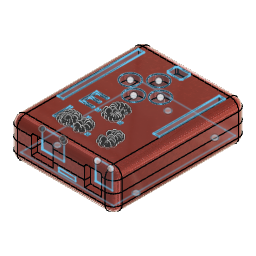
EdwinSolano_lab3_caja (Autodesk Fusion 360 design; units mm, degrees)
Autodesk Fusion 360 part; units mm, degrees
note: some values were not read from the file. Set by a fixed rule: which face or edge a step refers to.
sketch "sketch 1624" plane through (0, 0, 0) normal (0, 0, 1) x (1, 0, 0)
  line L0 (-54.34, 66.04) -> (-54.34, 0)
  line L1 (-54.34, 0) -> (-54.34, -3)
  line L2 (-54.34, -3) -> (-53.34, -3)
  line L3 (-53.34, -3) -> (0, -3)
  line L4 (0, -3) -> (1, -3)
  line L5 (1, -3) -> (1, 0)
  line L6 (1, 0) -> (1, 66.04)
  line L7 (1, 69.58) -> (1, 66.04)
  line L8 (-5.08, 69.58) -> (1, 69.58)
  line L9 (-5.08, 69.58) -> (-37.846, 69.58)
  line L10 (-54.34, 69.58) -> (-37.846, 69.58)
  line L11 (-54.34, 66.04) -> (-54.34, 69.58)
extrude "Extrude1" add sketch "sketch 1624" along normal blind 16.5 makes body 1
fillet "Fillet1" radius 1.5 11 edges at (-54.34, 33.29, 16.5) (-53.84, -3, 16.5) (-26.17, -3, 16.5) (1, 33.29, 16.5) (-26.67, 69.58, 16.5) (-54.34, 69.58, 8.25) (-54.34, -3, 8.25) (1, -3, 8.25) (-53.84, -3, 0) (-26.17, -3, 0) (-54.34, 33.29, 0) on bodies 1
fillet "Fillet2" radius 1.5 6 edges at (0.5607, -2.5607, 0.4393) (1, 34.04, 0) (1, 69.58, 7.5) (0.5607, 69.1407, 16.0607) (-53.9007, 69.1407, 0.4393) (-25.92, 69.58, 0) on bodies 1
shell "Shell1" thickness 3.6 outward yes removed faces 0 bodies 1
ref_plane "WorkPlane1" through (-26.67, 33.29, 8.25) normal (0, 0, 1) x (1, 0, 0)
split "Split1" by plane through (-26.67, 33.29, 8.25) normal (0, 0, 1) bodies 1 makes body 2 at (-35.3933, 21.6933, 20.1)
copy_body "Body->Comp1" bodies 2 removing the originals makes body 3 in component "parteArriba"
copy_body "Body->Comp2" bodies 1 removing the originals makes body 4 in component "parteAbajo"
sketch "sketch 1670" plane through (0, 0, 0) normal (0, -1, 0) x (1, 0, 0)
  spline S0 degree 3 poles (-31.5, 15.59) (-31.5, 15.7159) (-31.5248, 15.8406) (-31.5729, 15.9569) (-31.6211, 16.0735) (-31.6918, 16.1794) (-31.7809, 16.2686) (-31.8701, 16.3578) (-31.9759, 16.4286) (-32.0924, 16.4768) (-32.209, 16.5251) (-32.3339, 16.55) (-32.46, 16.55) knots -0.073178 -0.073178 -0.073178 -0.073178 -0.054906 -0.054906 -0.054906 -0.036606 -0.036606 -0.036606 -0.018305 -0.018305 -0.018305 0 0 0 0
  line L0 (-32.46, 16.55) -> (-43.58, 16.55)
  spline S1 degree 3 poles (-43.58, 16.55) (-43.7059, 16.55) (-43.8306, 16.5252) (-43.9469, 16.4771) (-44.0635, 16.4289) (-44.1694, 16.3582) (-44.2586, 16.2691) (-44.3478, 16.1799) (-44.4186, 16.0741) (-44.4668, 15.9576) (-44.5151, 15.841) (-44.54, 15.7161) (-44.54, 15.59) knots -0.073178 -0.073178 -0.073178 -0.073178 -0.054906 -0.054906 -0.054906 -0.036606 -0.036606 -0.036606 -0.018305 -0.018305 -0.018305 0 0 0 0
  line L1 (-44.54, 15.59) -> (-44.54, 15.49)
  line L2 (-44.54, 15.49) -> (-44.54, 5.84)
  line L3 (-44.54, 5.84) -> (-44.54, 5)
  line L4 (-31.5, 5) -> (-44.54, 5)
  line L5 (-31.5, 5) -> (-31.5, 5.84)
  line L6 (-31.5, 5.84) -> (-31.5, 15.49)
  line L7 (-31.5, 15.59) -> (-31.5, 15.49)
  arc A0 (-11.675, 16.5) -> (-12.675, 15.5) centre (-11.675, 15.5) ccw
  line L8 (-12.675, 15.5) -> (-12.675, 4.5)
  line L9 (-12.675, 4.5) -> (-2.675, 4.5)
  line L10 (-2.675, 4.5) -> (-2.675, 15.5)
  arc A1 (-2.675, 15.5) -> (-3.675, 16.5) centre (-3.675, 15.5) ccw
  line L11 (-3.675, 16.5) -> (-11.675, 16.5)
extrude "Extrude1'" cut sketch "sketch 1670" along normal up to surface (6.6 mm away) bodies 3 in component "parteArriba"
sketch "sketch 1744" plane through (0, 0, 0) normal (0, -1, 0) x (1, 0, 0)
  spline S0 degree 3 poles (-31.5, 15.59) (-31.5, 15.7159) (-31.5248, 15.8406) (-31.5729, 15.9569) (-31.6211, 16.0735) (-31.6918, 16.1794) (-31.7809, 16.2686) (-31.8701, 16.3578) (-31.9759, 16.4286) (-32.0924, 16.4768) (-32.209, 16.5251) (-32.3339, 16.55) (-32.46, 16.55) knots -0.073178 -0.073178 -0.073178 -0.073178 -0.054906 -0.054906 -0.054906 -0.036606 -0.036606 -0.036606 -0.018305 -0.018305 -0.018305 0 0 0 0
  line L0 (-32.46, 16.55) -> (-43.58, 16.55)
  spline S1 degree 3 poles (-43.58, 16.55) (-43.7059, 16.55) (-43.8306, 16.5252) (-43.9469, 16.4771) (-44.0635, 16.4289) (-44.1694, 16.3582) (-44.2586, 16.2691) (-44.3478, 16.1799) (-44.4186, 16.0741) (-44.4668, 15.9576) (-44.5151, 15.841) (-44.54, 15.7161) (-44.54, 15.59) knots -0.073178 -0.073178 -0.073178 -0.073178 -0.054906 -0.054906 -0.054906 -0.036606 -0.036606 -0.036606 -0.018305 -0.018305 -0.018305 0 0 0 0
  line L1 (-44.54, 15.59) -> (-44.54, 15.49)
  line L2 (-44.54, 15.49) -> (-44.54, 5.84)
  line L3 (-44.54, 5.84) -> (-44.54, 5)
  line L4 (-31.5, 5) -> (-44.54, 5)
  line L5 (-31.5, 5) -> (-31.5, 5.84)
  line L6 (-31.5, 5.84) -> (-31.5, 15.49)
  line L7 (-31.5, 15.59) -> (-31.5, 15.49)
  arc A0 (-11.675, 16.5) -> (-12.675, 15.5) centre (-11.675, 15.5) ccw
  line L8 (-12.675, 15.5) -> (-12.675, 4.5)
  line L9 (-12.675, 4.5) -> (-2.675, 4.5)
  line L10 (-2.675, 4.5) -> (-2.675, 15.5)
  arc A1 (-2.675, 15.5) -> (-3.675, 16.5) centre (-3.675, 15.5) ccw
  line L11 (-3.675, 16.5) -> (-11.675, 16.5)
extrude "Extrude1''" cut sketch "sketch 1744" along normal up to surface (6.6 mm away) bodies 4 in component "parteAbajo"
sketch "sketch 1818" plane through (0, 0, 20.1) normal (0, 0, 1) x (-1, 0, 0)
  line L0 (32.2, -62.7029) -> (32.2, -67.1171)
  line L1 (31.4071, -61.91) -> (32.2, -62.7029)
  line L2 (24.3729, -61.91) -> (31.4071, -61.91)
  line L3 (23.58, -62.7029) -> (24.3729, -61.91)
  line L4 (23.58, -67.1171) -> (23.58, -62.7029)
  line L5 (24.3729, -67.91) -> (23.58, -67.1171)
  line L6 (31.4071, -67.91) -> (24.3729, -67.91)
  line L7 (32.2, -67.1171) -> (31.4071, -67.91)
  line L8 (49.095, -65.27) -> (49.095, -17.026)
  line L9 (52.505, -65.27) -> (49.095, -65.27)
  line L10 (52.505, -17.026) -> (52.505, -65.27)
  line L11 (49.095, -17.026) -> (52.505, -17.026)
  line L12 (0.835, -65.27) -> (0.835, -26.17)
  line L13 (4.245, -65.27) -> (0.835, -65.27)
  line L14 (4.245, -26.17) -> (4.245, -65.27)
  line L15 (0.835, -26.17) -> (4.245, -26.17)
extrude "Extrude2" cut sketch "sketch 1818" against normal up to surface (23.7 mm away) bodies 3 in component "parteArriba"
sketch "sketch 1883" plane through (0, 0, 20.1) normal (0, 0, 1) x (-1, 0, 0)
  line L0 (32.2, -62.7029) -> (32.2, -67.1171)
  line L1 (31.4071, -61.91) -> (32.2, -62.7029)
  line L2 (24.3729, -61.91) -> (31.4071, -61.91)
  line L3 (23.58, -62.7029) -> (24.3729, -61.91)
  line L4 (23.58, -67.1171) -> (23.58, -62.7029)
  line L5 (24.3729, -67.91) -> (23.58, -67.1171)
  line L6 (31.4071, -67.91) -> (24.3729, -67.91)
  line L7 (32.2, -67.1171) -> (31.4071, -67.91)
  line L8 (49.095, -65.27) -> (49.095, -17.026)
  line L9 (52.505, -65.27) -> (49.095, -65.27)
  line L10 (52.505, -17.026) -> (52.505, -65.27)
  line L11 (49.095, -17.026) -> (52.505, -17.026)
  line L12 (0.835, -65.27) -> (0.835, -26.17)
  line L13 (4.245, -65.27) -> (0.835, -65.27)
  line L14 (4.245, -26.17) -> (4.245, -65.27)
  line L15 (0.835, -26.17) -> (4.245, -26.17)
extrude "Extrude2'" cut sketch "sketch 1883" against normal up to surface (23.7 mm away) bodies 4 in component "parteAbajo"
sketch "sketch 1948" plane through (0, -6.6, 0) normal (0, -1, 0) x (1, 0, 0)
  line L0 (-18, 5) -> (-28, 5)
  line L1 (-18, 7) -> (-18, 5)
  line L2 (-28, 7) -> (-18, 7)
  line L3 (-28, 5) -> (-28, 7)
extrude "Extrude3" cut sketch "sketch 1948" along normal blind 0.8 from surface at -3.6 bodies 4 in component "parteAbajo"
sketch "sketch 1975" plane through (0, 0, 20.1) normal (0, 0, 1) x (-1, 0, 0)
  line L0 (23.0486, -5.5376) -> (24.447, -5.5376)
  line L1 (23.0486, -6.936) -> (23.0486, -5.5376)
  line L2 (24.447, -6.936) -> (23.0486, -6.936)
  line L3 (24.447, -5.5376) -> (24.447, -6.936)
  line L4 (31.432, -6.4448) -> (31.432, -5.5376)
  spline S0 degree 3 poles (29.4197, -5.3739) (29.8245, -5.4191) (30.6367, -5.5097) (31.1663, -6.1325) (31.432, -6.4448) knots 0 0 0 0 0.117517 0.235779 0.235779 0.235779 0.235779
  spline S1 degree 3 poles (27.2096, -6.3902) (27.528, -6.0938) (28.1537, -5.5113) (29.0027, -5.4191) (29.4197, -5.3739) knots 0 0 0 0 0.126774 0.249154 0.249154 0.249154 0.249154
  spline S2 degree 3 poles (26.2887, -9.2688) (26.3125, -8.7007) (26.3562, -7.6523) (26.9415, -6.7867) (27.2096, -6.3902) knots 0 0 0 0 0.166672 0.307547 0.307547 0.307547 0.307547
  spline S3 degree 3 poles (26.507, -10.7422) (26.4434, -10.506) (26.3133, -10.0234) (26.297, -9.5238) (26.2887, -9.2688) knots 0 0 0 0 0.073138 0.149391 0.149391 0.149391 0.149391
  spline S4 degree 3 poles (27.1107, -11.9189) (26.9879, -11.7438) (26.7325, -11.3796) (26.5841, -10.9601) (26.507, -10.7422) knots 0 0 0 0 0.06384 0.132796 0.132796 0.132796 0.132796
  spline S5 degree 3 poles (28.093, -12.6761) (27.9037, -12.5783) (27.5303, -12.3854) (27.2493, -12.073) (27.1107, -11.9189) knots 0 0 0 0 0.063318 0.124937 0.124937 0.124937 0.124937
  spline S6 degree 3 poles (29.3583, -12.9455) (29.139, -12.9345) (28.7027, -12.9127) (28.2955, -12.7546) (28.093, -12.6761) knots 0 0 0 0 0.065406 0.130119 0.130119 0.130119 0.130119
  spline S7 degree 3 poles (31.3433, -11.9701) (31.0681, -12.2546) (30.523, -12.8182) (29.7441, -12.9033) (29.3583, -12.9455) knots 0 0 0 0 0.114828 0.227492 0.227492 0.227492 0.227492
  line L5 (31.3433, -15.5376) -> (31.3433, -11.9701)
  line L6 (32.5711, -15.5376) -> (31.3433, -15.5376)
  line L7 (32.5711, -5.5376) -> (32.5711, -15.5376)
  line L8 (31.432, -5.5376) -> (32.5711, -5.5376)
  spline S8 degree 3 poles (30.859, -11.2368) (31.0296, -10.9591) (31.409, -10.3418) (31.4326, -9.6145) (31.4456, -9.2143) knots 0 0 0 0 0.096175 0.213822 0.213822 0.213822 0.213822
  spline S9 degree 3 poles (29.4674, -11.936) (29.7299, -11.9028) (30.2746, -11.8341) (30.6595, -11.4406) (30.859, -11.2368) knots 0 0 0 0 0.077043 0.159875 0.159875 0.159875 0.159875
  spline S10 degree 3 poles (28.1066, -11.2606) (28.3001, -11.4576) (28.6765, -11.8407) (29.2088, -11.9048) (29.4674, -11.936) knots 0 0 0 0 0.080181 0.15601 0.15601 0.15601 0.15601
  spline S11 degree 3 poles (27.5438, -9.1665) (27.5526, -9.5886) (27.5682, -10.337) (27.9431, -10.9802) (28.1066, -11.2606) knots 0 0 0 0 0.124095 0.22 0.22 0.22 0.22
  spline S12 degree 3 poles (28.1305, -7.0826) (27.9599, -7.3656) (27.5757, -8.003) (27.5552, -8.7507) (27.5438, -9.1665) knots 0 0 0 0 0.097543 0.219759 0.219759 0.219759 0.219759
  spline S13 degree 3 poles (29.522, -6.3834) (29.2595, -6.4166) (28.7149, -6.4853) (28.3299, -6.8788) (28.1305, -7.0826) knots 0 0 0 0 0.077043 0.159875 0.159875 0.159875 0.159875
  spline S14 degree 3 poles (31.0909, -7.3316) (30.8868, -7.0551) (30.4926, -6.5212) (29.8378, -6.4282) (29.522, -6.3834) knots 0 0 0 0 0.098539 0.190329 0.190329 0.190329 0.190329
  spline S15 degree 3 poles (31.4456, -9.2143) (31.4435, -8.8344) (31.44, -8.1827) (31.1937, -7.5821) (31.0909, -7.3316) knots 0 0 0 0 0.11256 0.193136 0.193136 0.193136 0.193136
  spline S16 degree 3 poles (35.361, -5.5376) (35.4194, -5.674) (35.5419, -5.9605) (35.5844, -6.2694) (35.6066, -6.4312) knots 0 0 0 0 0.04431 0.093043 0.093043 0.093043 0.093043
  line L9 (34.0786, -5.5376) -> (35.361, -5.5376)
  spline S17 degree 3 poles (34.389, -6.4073) (34.3561, -6.2571) (34.2898, -5.9539) (34.1494, -5.6772) (34.0786, -5.5376) knots 0 0 0 0 0.045934 0.092677 0.092677 0.092677 0.092677
  spline S18 degree 3 poles (34.4674, -8.5731) (34.4703, -8.1068) (34.4746, -7.3835) (34.4115, -6.6633) (34.389, -6.4073) knots 0 0 0 0 0.139765 0.216815 0.216815 0.216815 0.216815
  line L10 (34.4674, -10.2102) -> (34.4674, -8.5731)
  spline S19 degree 3 poles (34.5288, -11.3425) (34.5111, -11.196) (34.4657, -10.8201) (34.4668, -10.4413) (34.4674, -10.2102) knots 0 0 0 0 0.044238 0.11349 0.11349 0.11349 0.11349
  spline S20 degree 3 poles (34.9108, -12.1781) (34.8259, -12.0569) (34.6475, -11.802) (34.5697, -11.5005) (34.5288, -11.3425) knots 0 0 0 0 0.044035 0.092543 0.092543 0.092543 0.092543
  spline S21 degree 3 poles (35.7635, -12.7272) (35.5885, -12.6561) (35.2692, -12.5262) (35.0224, -12.2865) (34.9108, -12.1781) knots 0 0 0 0 0.056018 0.102261 0.102261 0.102261 0.102261
  spline S22 degree 3 poles (37.271, -12.9455) (36.9887, -12.9407) (36.4763, -12.9321) (35.9844, -12.7907) (35.7635, -12.7272) knots 0 0 0 0 0.084249 0.152908 0.152908 0.152908 0.152908
  spline S23 degree 3 poles (38.9149, -12.6897) (38.6614, -12.7642) (38.125, -12.922) (37.5659, -12.9374) (37.271, -12.9455) knots 0 0 0 0 0.078936 0.166992 0.166992 0.166992 0.166992
  spline S24 degree 3 poles (39.9995, -11.9598) (39.8543, -12.1109) (39.5459, -12.4318) (39.1333, -12.6005) (38.9149, -12.6897) knots 0 0 0 0 0.062163 0.132021 0.132021 0.132021 0.132021
  spline S25 degree 3 poles (40.5384, -10.7149) (40.4798, -10.9532) (40.3702, -11.3991) (40.1173, -11.7817) (39.9995, -11.9598) knots 0 0 0 0 0.072951 0.136549 0.136549 0.136549 0.136549
  line L11 (39.3378, -10.5512) -> (40.5384, -10.7149)
  spline S26 degree 3 poles (38.7273, -11.6256) (38.8588, -11.4925) (39.1569, -11.1907) (39.273, -10.7805) (39.3378, -10.5512) knots 0 0 0 0 0.055278 0.125347 0.125347 0.125347 0.125347
  spline S27 degree 3 poles (37.4483, -11.9291) (37.7049, -11.9251) (38.1557, -11.9181) (38.5552, -11.7137) (38.7273, -11.6256) knots 0 0 0 0 0.075671 0.132995 0.132995 0.132995 0.132995
  spline S28 degree 3 poles (36.05, -11.513) (36.2395, -11.634) (36.6636, -11.9047) (37.1689, -11.9204) (37.4483, -11.9291) knots 0 0 0 0 0.066297 0.148303 0.148303 0.148303 0.148303
  spline S29 degree 3 poles (35.7021, -10.4557) (35.707, -10.6776) (35.7156, -11.0688) (35.949, -11.3788) (36.05, -11.513) knots 0 0 0 0 0.064538 0.113796 0.113796 0.113796 0.113796
  spline S30 degree 3 poles (35.7089, -10.1351) (35.707, -10.2039) (35.704, -10.3108) (35.7026, -10.4176) (35.7021, -10.4557) knots 0 0 0 0 0.020641 0.032068 0.032068 0.032068 0.032068
  spline S31 degree 3 poles (37.8986, -9.7122) (37.4657, -9.7646) (36.7255, -9.8542) (36.0072, -10.0527) (35.7089, -10.1351) knots 0 0 0 0 0.130548 0.223278 0.223278 0.223278 0.223278
  spline S32 degree 3 poles (38.99, -9.528) (38.8391, -9.5613) (38.4785, -9.6409) (38.1118, -9.686) (37.8986, -9.7122) knots 0 0 0 0 0.046321 0.110737 0.110737 0.110737 0.110737
  spline S33 degree 3 poles (39.8733, -9.1256) (39.737, -9.2093) (39.4592, -9.3798) (39.1483, -9.478) (38.99, -9.528) knots 0 0 0 0 0.047794 0.097396 0.097396 0.097396 0.097396
  spline S34 degree 3 poles (40.5077, -8.4196) (40.4217, -8.5583) (40.2524, -8.8316) (39.9984, -9.0286) (39.8733, -9.1256) knots 0 0 0 0 0.04852 0.095596 0.095596 0.095596 0.095596
  spline S35 degree 3 poles (40.7498, -7.4475) (40.7404, -7.6199) (40.7217, -7.9595) (40.5783, -8.2678) (40.5077, -8.4196) knots 0 0 0 0 0.051263 0.100997 0.100997 0.100997 0.100997
  spline S36 degree 3 poles (40.1086, -5.9571) (40.2957, -6.1669) (40.6746, -6.5921) (40.7245, -7.1599) (40.7498, -7.4475) knots 0 0 0 0 0.082003 0.166167 0.166167 0.166167 0.166167
  spline S37 degree 3 poles (38.2737, -5.3739) (38.637, -5.3884) (39.3051, -5.4152) (39.8569, -5.7873) (40.1086, -5.9571) knots 0 0 0 0 0.106562 0.195931 0.195931 0.195931 0.195931
  spline S38 degree 3 poles (36.9197, -5.6126) (37.1359, -5.543) (37.5762, -5.4012) (38.0385, -5.3831) (38.2737, -5.3739) knots 0 0 0 0 0.067806 0.138063 0.138063 0.138063 0.138063
  spline S39 degree 3 poles (35.6066, -6.4312) (35.8231, -6.2556) (36.2271, -5.9279) (36.7002, -5.7126) (36.9197, -5.6126) knots 0 0 0 0 0.083222 0.155292 0.155292 0.155292 0.155292
  line L12 (35.7089, -8.7231) -> (35.7089, -9.1733)
  spline S40 degree 3 poles (35.9067, -7.4953) (35.8493, -7.6656) (35.7154, -8.0628) (35.7113, -8.483) (35.7089, -8.7231) knots 0 0 0 0 0.053595 0.125049 0.125049 0.125049 0.125049
  spline S41 degree 3 poles (36.7185, -6.646) (36.5472, -6.7576) (36.21, -6.9772) (36.0068, -7.3244) (35.9067, -7.4953) knots 0 0 0 0 0.060389 0.118927 0.118927 0.118927 0.118927
  spline S42 degree 3 poles (37.9804, -6.3357) (37.7534, -6.347) (37.3124, -6.369) (36.9125, -6.5555) (36.7185, -6.646) knots 0 0 0 0 0.067467 0.131055 0.131055 0.131055 0.131055
  spline S43 degree 3 poles (39.0684, -6.6631) (38.9201, -6.5678) (38.5904, -6.3561) (38.1969, -6.3429) (37.9804, -6.3357) knots 0 0 0 0 0.051957 0.115498 0.115498 0.115498 0.115498
  spline S44 degree 3 poles (39.4402, -7.4817) (39.4245, -7.3246) (39.3932, -7.0098) (39.1768, -6.7789) (39.0684, -6.6631) knots 0 0 0 0 0.04597 0.092167 0.092167 0.092167 0.092167
  spline S45 degree 3 poles (39.2696, -8.0649) (39.3194, -7.9746) (39.4195, -7.7929) (39.4332, -7.5858) (39.4402, -7.4817) knots 0 0 0 0 0.030521 0.061427 0.061427 0.061427 0.061427
  spline S46 degree 3 poles (38.7853, -8.4639) (38.8832, -8.4143) (39.0745, -8.3172) (39.2056, -8.1477) (39.2696, -8.0649) knots 0 0 0 0 0.032478 0.063457 0.063457 0.063457 0.063457
  spline S47 degree 3 poles (37.7144, -8.7095) (37.9316, -8.6784) (38.2958, -8.6262) (38.6446, -8.5106) (38.7853, -8.4639) knots 0 0 0 0 0.065664 0.11006 0.11006 0.11006 0.11006
  spline S48 degree 3 poles (35.7089, -9.1733) (35.9858, -9.0823) (36.6398, -8.8675) (37.3214, -8.7673) (37.7144, -8.7095) knots 0 0 0 0 0.087289 0.20617 0.20617 0.20617 0.20617
  line L13 (42.2369, -5.5376) -> (43.4647, -5.5376)
  line L14 (42.2369, -15.5376) -> (42.2369, -5.5376)
  line L15 (43.4647, -15.5376) -> (42.2369, -15.5376)
  line L16 (43.4647, -5.5376) -> (43.4647, -15.5376)
  spline S49 degree 3 poles (16.374, -6.1447) (16.6331, -6.4293) (17.1614, -7.0096) (17.2973, -7.7832) (17.3665, -8.1774) knots 0 0 0 0 0.113013 0.230401 0.230401 0.230401 0.230401
  spline S50 degree 3 poles (14.1878, -5.3602) (14.603, -5.3885) (15.4073, -5.4432) (16.0588, -5.916) (16.374, -6.1447) knots 0 0 0 0 0.122066 0.236492 0.236492 0.236492 0.236492
  spline S51 degree 3 poles (11.773, -6.2709) (12.1189, -6.0053) (12.8306, -5.4589) (13.727, -5.3937) (14.1878, -5.3602) knots 0 0 0 0 0.127883 0.263168 0.263168 0.263168 0.263168
  spline S52 degree 3 poles (10.8181, -8.4912) (10.8582, -8.0709) (10.9386, -7.2286) (11.4945, -6.5906) (11.773, -6.2709) knots 0 0 0 0 0.123325 0.247176 0.247176 0.247176 0.247176
  spline S53 degree 3 poles (11.3092, -10.1044) (11.166, -9.8689) (10.8652, -9.3741) (10.8343, -8.7948) (10.8181, -8.4912) knots 0 0 0 0 0.081376 0.170983 0.170983 0.170983 0.170983
  spline S54 degree 3 poles (12.6871, -10.9537) (12.4108, -10.8707) (11.8752, -10.7099) (11.4938, -10.302) (11.3092, -10.1044) knots 0 0 0 0 0.084836 0.164458 0.164458 0.164458 0.164458
  spline S55 degree 3 poles (11.6571, -11.7995) (11.7916, -11.6292) (12.073, -11.2728) (12.4765, -11.0631) (12.6871, -10.9537) knots 0 0 0 0 0.064354 0.134637 0.134637 0.134637 0.134637
  spline S56 degree 3 poles (11.3092, -12.9796) (11.3234, -12.7689) (11.3516, -12.3496) (11.5556, -11.9823) (11.6571, -11.7995) knots 0 0 0 0 0.062511 0.124386 0.124386 0.124386 0.124386
  spline S57 degree 3 poles (11.6741, -14.2688) (11.5677, -14.0645) (11.3569, -13.6598) (11.325, -13.2048) (11.3092, -12.9796) knots 0 0 0 0 0.068309 0.13527 0.13527 0.13527 0.13527
  spline S58 degree 3 poles (12.728, -15.2272) (12.5134, -15.1019) (12.0938, -14.857) (11.8118, -14.4618) (11.6741, -14.2688) knots 0 0 0 0 0.073622 0.143898 0.143898 0.143898 0.143898
  spline S59 degree 3 poles (14.2355, -15.5785) (13.9698, -15.5648) (13.4462, -15.5377) (12.965, -15.3297) (12.728, -15.2272) knots 0 0 0 0 0.079104 0.1559 0.1559 0.1559 0.1559
  spline S60 degree 3 poles (16.2205, -14.8998) (15.9319, -15.0977) (15.3343, -15.5075) (14.61, -15.5543) (14.2355, -15.5785) knots 0 0 0 0 0.102989 0.213272 0.213272 0.213272 0.213272
  spline S61 degree 3 poles (17.2437, -12.9864) (17.1519, -13.3686) (16.9769, -14.097) (16.4642, -14.6411) (16.2205, -14.8998) knots 0 0 0 0 0.115593 0.220352 0.220352 0.220352 0.220352
  line L17 (16.0159, -12.7681) -> (17.2437, -12.9864)
  spline S62 degree 3 poles (15.402, -14.1188) (15.5484, -13.9386) (15.8695, -13.5434) (15.9643, -13.0413) (16.0159, -12.7681) knots 0 0 0 0 0.068595 0.150441 0.150441 0.150441 0.150441
  spline S63 degree 3 poles (14.2082, -14.569) (14.435, -14.5521) (14.8777, -14.5192) (15.2301, -14.25) (15.402, -14.1188) knots 0 0 0 0 0.066613 0.130061 0.130061 0.130061 0.130061
  spline S64 degree 3 poles (13.0282, -14.1256) (13.1956, -14.2549) (13.5428, -14.5229) (13.9812, -14.5533) (14.2082, -14.569) knots 0 0 0 0 0.062022 0.128606 0.128606 0.128606 0.128606
  spline S65 degree 3 poles (12.5711, -13.0069) (12.5889, -13.2211) (12.6238, -13.6424) (12.8949, -13.9663) (13.0282, -14.1256) knots 0 0 0 0 0.062781 0.123515 0.123515 0.123515 0.123515
  spline S66 degree 3 poles (13.1987, -11.745) (13.0157, -11.905) (12.635, -12.2381) (12.593, -12.7441) (12.5711, -13.0069) knots 0 0 0 0 0.070147 0.145969 0.145969 0.145969 0.145969
  spline S67 degree 3 poles (14.6107, -11.3357) (14.3571, -11.3519) (13.8559, -11.3839) (13.416, -11.6256) (13.1987, -11.745) knots 0 0 0 0 0.075222 0.148626 0.148626 0.148626 0.148626
  spline S68 degree 3 poles (14.8085, -11.3493) (14.7716, -11.3454) (14.7058, -11.3383) (14.6397, -11.3365) (14.6107, -11.3357) knots 0 0 0 0 0.011132 0.019836 0.019836 0.019836 0.019836
  line L18 (14.9449, -10.2716) -> (14.8085, -11.3493)
  spline S69 degree 3 poles (14.0786, -10.408) (14.2093, -10.4002) (14.5023, -10.3828) (14.7872, -10.3112) (14.9449, -10.2716) knots 0 0 0 0 0.039201 0.087867 0.087867 0.087867 0.087867
  spline S70 degree 3 poles (12.6734, -9.8589) (12.8736, -10.019) (13.2842, -10.3476) (13.8094, -10.3875) (14.0786, -10.408) knots 0 0 0 0 0.075063 0.154028 0.154028 0.154028 0.154028
  spline S71 degree 3 poles (12.1209, -8.4639) (12.1417, -8.7313) (12.1824, -9.2539) (12.5123, -9.6603) (12.6734, -9.8589) knots 0 0 0 0 0.078392 0.15324 0.15324 0.15324 0.15324
  spline S72 degree 3 poles (12.7178, -6.9769) (12.5437, -7.1908) (12.191, -7.6243) (12.1445, -8.1816) (12.1209, -8.4639) knots 0 0 0 0 0.080736 0.163605 0.163605 0.163605 0.163605
  spline S73 degree 3 poles (14.181, -6.3766) (13.9041, -6.401) (13.3539, -6.4494) (12.9289, -6.8018) (12.7178, -6.9769) knots 0 0 0 0 0.081291 0.161533 0.161533 0.161533 0.161533
  spline S74 degree 3 poles (15.419, -6.837) (15.2383, -6.7028) (14.8707, -6.4295) (14.4135, -6.3944) (14.181, -6.3766) knots 0 0 0 0 0.066099 0.134519 0.134519 0.134519 0.134519
  spline S75 degree 3 poles (16.1387, -8.3411) (16.0679, -8.0296) (15.9411, -7.4715) (15.579, -7.0314) (15.419, -6.837) knots 0 0 0 0 0.094219 0.168777 0.168777 0.168777 0.168777
  line L19 (17.3665, -8.1774) -> (16.1387, -8.3411)
  line L20 (19.1741, -21.1447) -> (20.5725, -21.1447)
  line L21 (19.1741, -22.543) -> (19.1741, -21.1447)
  line L22 (20.5725, -22.543) -> (19.1741, -22.543)
  line L23 (20.5725, -21.1447) -> (20.5725, -22.543)
  spline S76 degree 3 poles (29.9825, -22.5601) (30.1358, -22.836) (30.447, -23.3957) (30.5031, -24.0339) (30.5316, -24.3575) knots 0 0 0 0 0.093565 0.189827 0.189827 0.189827 0.189827
  spline S77 degree 3 poles (28.5432, -21.3698) (28.8313, -21.5165) (29.4001, -21.8061) (29.79, -22.311) (29.9825, -22.5601) knots 0 0 0 0 0.095679 0.188858 0.188858 0.188858 0.188858
  spline S78 degree 3 poles (26.2683, -20.9741) (26.6881, -20.9848) (27.4669, -21.0046) (28.2036, -21.2546) (28.5432, -21.3698) knots 0 0 0 0 0.125136 0.23208 0.23208 0.23208 0.23208
  spline S79 degree 3 poles (24.3413, -21.3664) (24.6411, -21.252) (25.2615, -21.0154) (25.9253, -20.9882) (26.2683, -20.9741) knots 0 0 0 0 0.095616 0.19781 0.19781 0.19781 0.19781
  spline S80 degree 3 poles (23.0282, -22.4646) (23.2012, -22.2405) (23.5579, -21.7785) (24.075, -21.5065) (24.3413, -21.3664) knots 0 0 0 0 0.083895 0.172976 0.172976 0.172976 0.172976
  spline S81 degree 3 poles (22.5711, -23.9687) (22.5912, -23.7049) (22.6319, -23.1699) (22.8949, -22.7019) (23.0282, -22.4646) knots 0 0 0 0 0.078345 0.158903 0.158903 0.158903 0.158903
  spline S82 degree 3 poles (22.9872, -25.3909) (22.8659, -25.1746) (22.618, -24.7329) (22.587, -24.2269) (22.5711, -23.9687) knots 0 0 0 0 0.073388 0.1499 0.1499 0.1499 0.1499
  spline S83 degree 3 poles (24.2764, -26.4107) (24.01, -26.2754) (23.5106, -26.0219) (23.1537, -25.5916) (22.9872, -25.3909) knots 0 0 0 0 0.088542 0.165933 0.165933 0.165933 0.165933
  spline S84 degree 3 poles (26.49, -27.0485) (26.0331, -26.9464) (25.2819, -26.7786) (24.5595, -26.5143) (24.2764, -26.4107) knots 0 0 0 0 0.140231 0.230566 0.230566 0.230566 0.230566
  spline S85 degree 3 poles (28.4852, -27.7613) (28.2587, -27.6351) (27.6361, -27.2881) (26.9356, -27.1417) (26.49, -27.0485) knots 0 0 0 0 0.077449 0.212882 0.212882 0.212882 0.212882
  spline S86 degree 3 poles (28.874, -28.6481) (28.8584, -28.477) (28.8275, -28.1379) (28.5986, -27.8861) (28.4852, -27.7613) knots 0 0 0 0 0.050066 0.099215 0.099215 0.099215 0.099215
  spline S87 degree 3 poles (28.3249, -29.7088) (28.485, -29.5586) (28.7939, -29.2689) (28.848, -28.8499) (28.874, -28.6481) knots 0 0 0 0 0.063639 0.122808 0.122808 0.122808 0.122808
  spline S88 degree 3 poles (26.5752, -30.1488) (26.9298, -30.1434) (27.5509, -30.134) (28.0924, -29.8365) (28.3249, -29.7088) knots 0 0 0 0 0.10435 0.182822 0.182822 0.182822 0.182822
  spline S89 degree 3 poles (24.8324, -29.6645) (25.0701, -29.8053) (25.6046, -30.122) (26.2287, -30.1392) (26.5752, -30.1488) knots 0 0 0 0 0.081603 0.183535 0.183535 0.183535 0.183535
  spline S90 degree 3 poles (24.14, -28.232) (24.1877, -28.5229) (24.2775, -29.0707) (24.6552, -29.4749) (24.8324, -29.6645) knots 0 0 0 0 0.086188 0.16231 0.16231 0.16231 0.16231
  line L24 (22.8713, -28.3275) -> (24.14, -28.232)
  spline S91 degree 3 poles (23.3624, -29.9032) (23.2276, -29.6615) (22.954, -29.1708) (22.8991, -28.6114) (22.8713, -28.3275) knots 0 0 0 0 0.082079 0.166634 0.166634 0.166634 0.166634
  spline S92 degree 3 poles (24.6687, -30.9571) (24.4041, -30.827) (23.8891, -30.5736) (23.5347, -30.1226) (23.3624, -29.9032) knots 0 0 0 0 0.087185 0.169761 0.169761 0.169761 0.169761
  spline S93 degree 3 poles (26.6298, -31.3152) (26.2777, -31.3034) (25.6058, -31.2808) (24.9709, -31.0615) (24.6687, -30.9571) knots 0 0 0 0 0.105004 0.200355 0.200355 0.200355 0.200355
  spline S94 degree 3 poles (28.4647, -30.9741) (28.1769, -31.0736) (27.5826, -31.279) (26.954, -31.3029) (26.6298, -31.3152) knots 0 0 0 0 0.090819 0.187546 0.187546 0.187546 0.187546
  spline S95 degree 3 poles (29.7198, -29.9748) (29.5557, -30.1828) (29.2158, -30.6134) (28.7207, -30.8512) (28.4647, -30.9741) knots 0 0 0 0 0.0784 0.162332 0.162332 0.162332 0.162332
  spline S96 degree 3 poles (30.1496, -28.5594) (30.131, -28.8088) (30.0934, -29.3125) (29.8452, -29.7526) (29.7198, -29.9748) knots 0 0 0 0 0.074027 0.149548 0.149548 0.149548 0.149548
  spline S97 degree 3 poles (29.7983, -27.3145) (29.9007, -27.5068) (30.1082, -27.8961) (30.1357, -28.3365) (30.1496, -28.5594) knots 0 0 0 0 0.064541 0.130697 0.130697 0.130697 0.130697
  spline S98 degree 3 poles (28.7307, -26.3834) (28.9507, -26.5105) (29.3679, -26.7515) (29.6601, -27.1338) (29.7983, -27.3145) knots 0 0 0 0 0.075321 0.1429 0.1429 0.1429 0.1429
  spline S99 degree 3 poles (26.8003, -25.7593) (27.1951, -25.8536) (27.8555, -26.0114) (28.4797, -26.2767) (28.7307, -26.3834) knots 0 0 0 0 0.121486 0.203186 0.203186 0.203186 0.203186
  spline S100 degree 3 poles (25.02, -25.2716) (25.2348, -25.3404) (25.8211, -25.5284) (26.4206, -25.6697) (26.8003, -25.7593) knots 0 0 0 0 0.067667 0.184654 0.184654 0.184654 0.184654
  spline S101 degree 3 poles (24.1196, -24.6815) (24.2346, -24.7973) (24.4924, -25.0566) (24.832, -25.1949) (25.02, -25.2716) knots 0 0 0 0 0.04849 0.108625 0.108625 0.108625 0.108625
  spline S102 degree 3 poles (23.8467, -23.8596) (23.8574, -24.0105) (23.8784, -24.308) (24.04, -24.5583) (24.1196, -24.6815) knots 0 0 0 0 0.044607 0.087867 0.087867 0.087867 0.087867
  spline S103 degree 3 poles (24.1298, -23.0035) (24.0472, -23.1363) (23.8839, -23.399) (23.859, -23.7072) (23.8467, -23.8596) knots 0 0 0 0 0.046182 0.091335 0.091335 0.091335 0.091335
  spline S104 degree 3 poles (24.9927, -22.3862) (24.8155, -22.4633) (24.4832, -22.6078) (24.2422, -22.8776) (24.1298, -23.0035) knots 0 0 0 0 0.057174 0.107219 0.107219 0.107219 0.107219
  spline S105 degree 3 poles (26.3297, -22.1611) (26.0901, -22.1684) (25.6338, -22.1824) (25.1991, -22.3205) (24.9927, -22.3862) knots 0 0 0 0 0.071504 0.136162 0.136162 0.136162 0.136162
  spline S106 degree 3 poles (27.8644, -22.4578) (27.6253, -22.3713) (27.1295, -22.1919) (26.6025, -22.1716) (26.3297, -22.1611) knots 0 0 0 0 0.075816 0.157158 0.157158 0.157158 0.157158
  spline S107 degree 3 poles (28.8706, -23.2354) (28.741, -23.08) (28.4635, -22.7473) (28.0727, -22.5584) (27.8644, -22.4578) knots 0 0 0 0 0.06001 0.128469 0.128469 0.128469 0.128469
  spline S108 degree 3 poles (29.2833, -24.4666) (29.2481, -24.2342) (29.1822, -23.7991) (28.9696, -23.4145) (28.8706, -23.2354) knots 0 0 0 0 0.069873 0.130775 0.130775 0.130775 0.130775
  line L25 (30.5316, -24.3575) -> (29.2833, -24.4666)
  line L26 (32.3733, -21.1447) -> (33.7717, -21.1447)
  line L27 (32.3733, -22.543) -> (32.3733, -21.1447)
  line L28 (33.7717, -22.543) -> (32.3733, -22.543)
  line L29 (33.7717, -21.1447) -> (33.7717, -22.543)
  line L30 (35.7908, -21.1447) -> (43.2533, -21.1447)
  line L31 (35.7908, -22.3248) -> (35.7908, -21.1447)
  line L32 (41.9299, -22.3248) -> (35.7908, -22.3248)
  line L33 (41.9299, -25.7286) -> (41.9299, -22.3248)
  line L34 (36.3979, -25.7286) -> (41.9299, -25.7286)
  line L35 (36.3979, -26.9018) -> (36.3979, -25.7286)
  line L36 (41.9299, -26.9018) -> (36.3979, -26.9018)
  line L37 (41.9299, -29.9646) -> (41.9299, -26.9018)
  line L38 (36.0227, -29.9646) -> (41.9299, -29.9646)
  line L39 (36.0227, -31.1447) -> (36.0227, -29.9646)
  line L40 (43.2533, -31.1447) -> (36.0227, -31.1447)
  line L41 (43.2533, -21.1447) -> (43.2533, -31.1447)
extrude "Extrude3'" cut sketch "sketch 1975" against normal blind 2 bodies 3 in component "parteArriba"
sketch "sketch 2778" plane through (0, 0, 20.1) normal (0, 0, 1) x (-1, 0, 0)
  circle A0 centre (30, -40) radius 5
  circle A1 centre (30, -55) radius 5
  circle A2 centre (21, -47) radius 5
  circle A3 centre (39, -47) radius 5
extrude "Extrude4" cut sketch "sketch 2778" against normal blind 5.5 bodies 3 in component "parteArriba"
sketch "sketch 2808" plane through (0, 0, -3.6) normal (0, 0, -1) x (1, 0, 0)
  circle A0 centre (-2.54, -13.97) radius 1.5875
  circle A1 centre (-35.56, -66.04) radius 1.5875
  circle A2 centre (-50.8, -15.24) radius 1.5875
  circle A3 centre (-7.62, -66.04) radius 1.5875
extrude "Extrude4'" add sketch "sketch 2808" against normal blind 9 bodies 4 in component "parteAbajo"
component "parteArriba" placed x (1, 0, 0) y (0, 1, 0) z (0, 0, 1) at (0, 0, 0)
component "parteAbajo" placed x (1, 0, 0) y (0, 1, 0) z (0, 0, 1) at (0, 0, 0)
